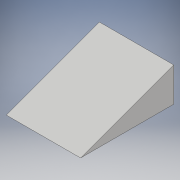
# Autodesk Inventor part: 70DegreeWoodHinge
Saved by Autodesk Inventor 2017 (Build 210142000, 142)
## iProperties
Created: 2017-11-02
Part Number: 70DegreeWoodHinge
Material: Generic
Document SubType Name: Modeling
Designer: Aidan_Moga
Density: 1 g/cm^3
Appearance: Default
Mass: 15.8001 g
Surface Area: 52.4561 cm^2
Volume: 15.8001 cm^3
Author: Aidan_Moga
Autodesk Inventor part; units mm, degrees
ref_plane "YZ Plane" through (0, 0, 0) normal (1, 0, 0) x (0, 1, 0)
ref_plane "XZ Plane" through (0, 0, 0) normal (0, 1, 0) x (-1, 0, 0)
ref_plane "XY Plane" through (0, 0, 0) normal (0, 0, 1) x (1, 0, 0)
sketch "Sketch1" plane through (0, 0, 0) normal (0, 0, 1) x (1, 0, 0)
  line L0 (38.1, 0) -> (-9.6364, 17.3746)
  line L1 (-9.6364, 17.3746) -> (-9.6364, 0)
  line L2 (-9.6364, 0) -> (38.1, 0)
  point P0 (0, 0)
  dimension "d2" = 50.8
  dimension "d4" = 70
  constraints: 6 end point, 1 horizontal, 1 vertical
  measures "d2" distance of L0.start L0.end
  measures "d4" angle of L1 L0
extrude "Extrusion1" add sketch "Sketch1" along normal blind 38.1
move or copy body "Move Body1" bodies to move or copy 1 copy no rotation origin (0, 0, 0) rotation axis (0, 1, 0) rotation angle -180 translate (-19.2728, 0, 76.2)
move or copy body "Move Body2" bodies to move or copy 1 copy no rotation origin (0, 0, 0) rotation axis (0, 1, 0) rotation angle 90 translate (-85.8364, 0, 66.5636)
body "Solid1"
